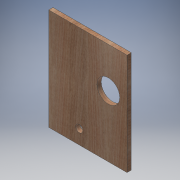
# Autodesk Inventor part: cannonSideWall
Saved by Autodesk Inventor 2018 (Build 220112000, 112)
## iProperties
Created: 2017-05-03
Part Number: cannonSideWall
Material: Generic
Document SubType Name: Modeling
Designer: gsegs
Density: 1 g/cm^3
Appearance: Birch - Natural Polished
Author: gsegs
Autodesk Inventor part; units mm, degrees
ref_plane "YZ Plane" through (0, 0, 0) normal (1, 0, 0) x (0, 1, 0)
ref_plane "XZ Plane" through (0, 0, 0) normal (0, 1, 0) x (-1, 0, 0)
ref_plane "Work Plane1" through (-4668.2945, 0, 0) normal (0, 0, 1) x (1, 0, 0)
sketch "Sketch1" plane through (-4668.2945, 0, 0) normal (0, 0, 1) x (1, 0, 0)
  line L0 (0, 19.05) -> (466.725, 19.05) projected
  line L1 (466.725, 0) -> (466.725, 19.05) projected
  line L2 (0, 0) -> (0, 19.05) projected
  line L3 (0, -340.481) -> (0, -321.431) projected
  line L4 (466.725, -340.481) -> (0, -340.481) projected
  line L5 (466.725, -340.481) -> (0, -340.481) projected
  line L6 (466.725, -340.481) -> (466.725, -321.431) projected
  line L7 (0, -321.431) -> (466.725, -321.431) construction
  line L8 (0, -340.481) -> (0, -321.431) projected
  line L9 (466.725, 19.05) -> (0, 19.05)
  line L10 (0, 19.05) -> (0, -340.481) construction
  line L11 (466.725, -340.481) -> (466.725, 19.05) construction
  line L12 (147.3639, -408.7465) -> (46.3111, -408.7465) construction
  line L13 (466.725, -340.481) -> (466.725, -408.7465) construction
  line L14 (466.725, -408.7465) -> (147.3639, -408.7465) construction
  line L15 (46.3111, -408.7465) -> (0, -408.7465)
  line L16 (0, -408.7465) -> (0, -340.481) construction
  line L17 (466.725, -408.7465) -> (466.725, -434.1465)
  line L18 (466.725, -434.1465) -> (0, -434.1465)
  line L19 (0, -434.1465) -> (0, -408.7465)
  line L20 (400.05, 19.05) -> (400.05, 0)
  line L21 (400.05, -321.431) -> (400.05, -340.481)
  line L22 (400.05, 0) -> (400.05, -321.431)
  line L23 (400.05, -340.481) -> (400.05, -434.1465)
  line L24 (101.6, 19.05) -> (101.6, 0)
  line L25 (101.6, -321.431) -> (101.6, -340.481)
  line L26 (101.6, 0) -> (101.6, -321.431)
  line L27 (101.6, -340.481) -> (101.6, -434.1465)
  point P0 (4668.2945, 0)
  point P1 (50.8, 19.05)
  point P2 (50.8, -321.431)
  point P3 (50.8, -340.481)
  point P4 (50.8, -434.1465)
  dimension "d7" = 25.4
  constraints: 38 end point, 8 perpendicular, 7 vertical, 3 horizontal, 3 point on line, 1 parallel, 13 other
  measures "d7" distance of L13.end L17.end
extrude "Extrusion1" add sketch "Sketch1" along normal blind 19.05
sketch "Sketch2" plane through (-4668.2945, 0, 0) normal (0, 0, -1) x (-1, 0, 0)
  line L0 (-232.5687, -355.978) -> (-232.5688, 34.547)
  line L1 (-141.2875, -408.7465) -> (-141.2875, 124.6535)
  circle A0 centre (-186.9249, -370.6465) radius 15.875
  line L2 (-232.5687, -370.6465) -> (-141.2875, -370.6465) construction
  line L3 (0, -408.7465) -> (-466.725, -408.7465) projected
  point P0 (-4668.2945, 0)
  dimension "d2" = 31.75
  dimension "d3" = 45.6438
  dimension "d4" = 38.1
  constraints: 6 end point, 3 point on line, 2 vertical, 1 centre point, 1 perpendicular, 4 other
  measures "d2" diameter of A0
  measures "d3" distance from line of L0 A0.centre
  measures "d4" distance between parallel lines of L3 L2
extrude "Extrusion2" cut sketch "Sketch2" against normal up to next
sketch "Sketch3" plane through (-4668.2945, 0, 0) normal (0, 0, -1) x (-1, 0, 0)
  circle A0 centre (-186.9249, -370.6465) radius 15.875 projected
  arc A1 (-207.9625, -430.5603) -> (-155.5881, -425.8756) centre (-186.9249, -370.6465) ccw
  line L0 (-101.6, -434.1465) -> (-400.05, -434.1465) projected
  line L1 (0, -340.481) -> (-157.1625, -426.7397)
  line L2 (-466.725, -340.481) -> (-207.9625, -430.5603)
  line L3 (-466.725, -434.1465) -> (-466.725, -340.481)
  line L4 (-466.725, -434.1465) -> (-466.725, 19.05) projected
  line L5 (-101.6, -434.1465) -> (-400.05, -434.1465) projected
  line L6 (0, -434.1465) -> (0, -340.481)
  line L7 (0, 19.05) -> (0, -434.1465) projected
  arc A2 (-155.5881, -425.8756) -> (-207.9625, -430.5603) centre (-186.9249, -370.6465) ccw construction
  line L8 (-101.6, 19.05) -> (-101.6, -434.1465) projected
  line L9 (-101.6, -396.2442) -> (-101.6, -434.1465)
  line L10 (-400.05, -434.1465) -> (-400.05, 19.05) projected
  line L11 (-400.05, -363.6916) -> (-400.05, -434.1465)
  point P0 (-4668.2945, 0)
  point P1 (-186.9249, -434.1465)
  point P2 (-50.8, -434.1465)
  constraints: 12 end point, 6 point on circle, 5 point on line, 3 collinear, 2 centre point, 1 vertical, 2 other
extrude "Extrusion3" cut sketch "Sketch3" against normal blind 19.05
sketch "Sketch4" plane through (-4668.2945, 0, 19.05) normal (0, 0, 1) x (1, 0, 0)
  circle A0 centre (316.7063, -160.7155) radius 12.7 construction
  circle A1 centre (316.7063, -160.7155) radius 50.8
  point P0 (4668.2945, 0)
  dimension "d10" = 101.6
  constraints: 1 centre point, 1 coincident
  measures "d10" diameter of A1
extrude "Extrusion4" cut sketch "Sketch4" against normal up to next
body "Solid1"
